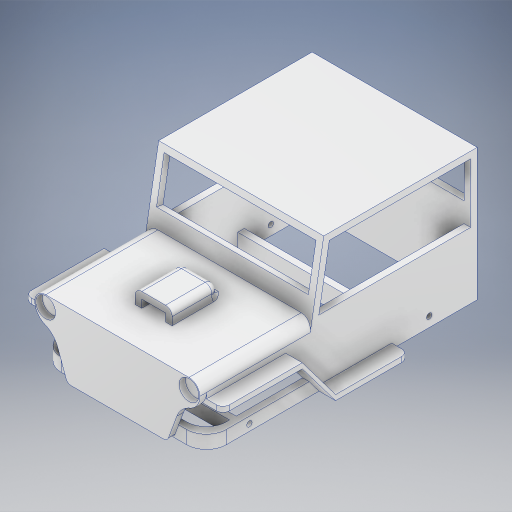
# Autodesk Inventor part: shell
Saved by Autodesk Inventor 2024 (Build 280153000, 153)
## iProperties
Created: 2024-04-09
Part Number: shell
Material: Aluminum 6061
Document SubType Name: Modeling
Designer: Alex
Density: 2.7 g/cm^3
Appearance: Aluminum - Flat
Mass: 9349.95 g
Surface Area: 5768.37 cm^2
Volume: 3462.95 cm^3
Author: Alex
Autodesk Inventor part; units mm, degrees
sketch "Sketch1" plane through (0, 0, 0) normal (1, 0, 0) x (0, 1, 0)
  line L0 (0, 0) -> (100, 0)
  line L1 (100, 0) -> (100, -160)
  line L2 (100, -410) -> (0, -410)
  line L3 (0, -410) -> (0, -400) construction
  line L4 (0, -410) -> (0, -410) construction
  line L5 (200, -410) -> (200, -177.6327)
  line L6 (200, -160) -> (100, -160) construction
  line L7 (100, -160) -> (0, -160) construction
  line L8 (100, -160) -> (100, -410) construction
  circle A0 centre (0, -50) radius 60 construction
  arc A1 (0, -400) -> (0, -280) centre (0, -340) ccw
  line L9 (0, -410) -> (24.2501, -410)
  line L10 (0, -393.7256) -> (0, -400)
  line L11 (0, -400) -> (0, -410)
  line L12 (0, -410) -> (200, -410)
  line L13 (0, -400) -> (0, -410)
  line L14 (0, -400) -> (0, 0) construction
  line L15 (0, -400) -> (0, -410)
  arc A2 (0, -400) -> (0, -400) centre (0, -340) ccw construction
  arc A3 (0, -280) -> (0, -400) centre (0, -340) ccw construction
  line L16 (0, -280) -> (0, -400) construction
  line L17 (0, -110) -> (0, -280)
  line L18 (75, 0) -> (67, 0)
  line L19 (67, 0) -> (67, -120)
  line L20 (67, -120) -> (75, -120) construction
  line L21 (75, -120) -> (75, 0)
  line L22 (8, -170.5357) -> (0, -170.5357) construction
  line L23 (0, -170.5357) -> (0, -280)
  line L24 (0, -280.5357) -> (8, -280.5357) construction
  line L25 (8, -280.5357) -> (8, -170.5357)
  line L26 (75, -120) -> (8, -170.5357)
  line L27 (67, -120) -> (0, -170.5357)
  line L28 (0, -280) -> (0, -280.5357) construction
  line L29 (100, -160) -> (200, -177.6327)
  line L30 (200, -177.6327) -> (200, -160) construction
  point P0 (67, 0)
  point P1 (0, -170.5357)
  dimension "d5" = 120
  dimension "d0" = 100
  dimension "d1" = 410
  dimension "d2" = 200
  dimension "d3" = 250
  dimension "d4" = 50
  dimension "d6" = 70
  dimension "d8" = 8
  dimension "d9" = 8
  dimension "d12" = 25
  dimension "d13" = 110
  dimension "d14" = 120
  dimension "d25" = 10
  dimension "d41" = 10
  constraints: 62 end point, 18 parallel, 10 perpendicular, 7 point on circle, 6 horizontal, 6 point on line, 3 centre point, 3 collinear, 1 midpoint, 1 vertical alignment, 3 other
  measures "d0" distance of L2.start L2.end
  measures "d1" distance of L0.end L2.start
  measures "d2" distance of L7.end L6.start
  measures "d3" distance of L6.start L5.start
  measures "d4" distance from line of point (0, -50) L0
  measures "d6" distance from line of L2 A1.centre
  measures "d8" distance of L19.end L20.end
  measures "d9" distance of L22.start L22.end
  measures "d12" distance between parallel lines of L21 L1
  measures "d13" distance of L24.end L22.start
  measures "d14" distance of L20.end L18.start
  measures "d25" angle of L29 L6
  measures "d41" distance of L11.start L4.end
extrude "Extrusion1" add sketch "Sketch1" against normal blind 250
sketch "Sketch2" plane through (0, 67, 0) normal (0, 0, 1) x (1, 0, 0)
  line L0 (-250, 33) -> (-250, 140.3403) projected
  line L1 (-250, 33) -> (0, 33)
  line L2 (0, 33) -> (0, -67) construction
  line L3 (-250, -67) -> (-250, 33) construction
  circle A0 centre (-233.5, 16.5) radius 15
  circle A1 centre (-16.5, 16.5) radius 15
  line L4 (0, 33) -> (0, 0) construction
  line L5 (0, 33) -> (-250, 33) construction
  line L6 (-250, 0) -> (-250, 33) construction
  line L7 (0, 0) -> (-250, 0) construction
  line L8 (-250, 16.5) -> (0, 16.5) construction
  arc A2 (-233.5, 33) -> (-250, 16.5) centre (-233.5, 16.5) ccw
  line L9 (0, 33) -> (-250, 33) projected
  line L10 (-250, 0) -> (-250, 33) projected
  arc A3 (0, 16.5) -> (-16.5, 33) centre (-16.5, 16.5) ccw
  line L11 (0, 33) -> (0, 0) projected
  arc A4 (-250, 16.5) -> (-234.6174, -6.5761) centre (-225, 16.5) ccw
  arc A5 (-215.1925, -26.9119) -> (-234.6174, -6.5761) centre (-248.0818, -38.8826) ccw
  line L12 (-215.1925, -26.9119) -> (-202.5175, -61.7362)
  arc A6 (-202.5175, -61.7362) -> (-195, -67) centre (-195, -59) ccw
  line L13 (-195, -67) -> (-55, -67)
  arc A7 (-55, -67) -> (-47.4825, -61.7362) centre (-55, -59) ccw
  line L14 (-47.4825, -61.7362) -> (-34.8075, -26.9119)
  arc A8 (-15.3826, -6.5761) -> (-34.8075, -26.9119) centre (-1.9182, -38.8826) ccw
  arc A9 (-15.3826, -6.5761) -> (0, 16.5) centre (-25, 16.5) ccw
  line L15 (-125, 16.5) -> (-125, -67) construction
  line L16 (0, -67) -> (-250, -67) construction
  line L17 (-250, -67) -> (0, -67) construction
  line L18 (0, 0) -> (-250, 0) projected
  line L19 (-6.2184, 0) -> (0, 0)
  line L20 (0, 0) -> (0, 16.5)
  line L21 (-243.7816, 0) -> (-250, 0)
  line L22 (-250, 0) -> (-250, 16.5)
  dimension "d17" = 30
  dimension "d18" = 25
  dimension "d19" = 8
  dimension "d20" = 35
  dimension "d21" = 140
  dimension "d22" = 110
  constraints: 26 end point, 18 point on circle, 16 tangent, 10 centre point, 6 point on line, 5 collinear, 5 midpoint, 4 equal radius, 2 concentric, 2 horizontal, 2 perpendicular, 1 equal length, 1 parallel, 1 vertical
  measures "d17" diameter of A1
  measures "d18" radius of A4
  measures "d19" radius of A6
  measures "d20" radius of A5
  measures "d21" distance of L13.start L13.end
  measures "d22" angle of L13 L12
extrude "Extrusion2" add sketch "Sketch2" along normal blind 10 contours L1 A3 A9 L18 A4 A2 | L18 A9 A8 L14 A7 L13 A6 L12 A5 A4
extrude "Extrusion3" cut sketch "Sketch2" against normal up to surface contours L1 A2 L10 | L1 L11 A3 surface through (0, 100, -160) normal (0, 0.1736482, 0.9848078)
extrude "Extrusion4" add sketch "Sketch1" along normal blind 25 contours L0 L21 L26 L25 A1 L17 L27 L19
ref_plane "Work Plane1" through (-125, 0, 0) normal (-1, 0, 0) x (0, 0, 1)
mirror "Mirror1" about plane through (-125, 0, 0) normal (-1, 0, 0) of "Extrusion4"
sketch "Sketch5" plane through (-125, 0, 0) normal (-1, 0, 0) x (0, 0, 1)
  line L0 (-120, 75) -> (0, 75) construction
  line L1 (0, 75) -> (0, 83.5) construction
  line L2 (-157.0906, 83.5) -> (0, 83.5) construction
  line L3 (-157.0906, 83.5) -> (-177.6327, 200) construction
  line L4 (-177.6327, 200) -> (-410, 200) construction
  line L5 (-410, 200) -> (-410, 0) construction
  line L6 (-410, 0) -> (-400, 0) construction
  arc A0 (-280.5357, 8) -> (-400, 0) centre (-340, 0) ccw construction
  line L7 (-280.5357, 8) -> (-170.5357, 8) construction
  line L8 (-170.5357, 8) -> (-120, 75) construction
  line L9 (-186.0237, 190) -> (-167.2449, 83.5)
  line L10 (-186.0237, 190) -> (-400, 190)
  line L11 (-400, 190) -> (-400, 0)
  line L12 (-157.0906, 83.5) -> (-410, 83.5) construction
  line L13 (-167.2449, 83.5) -> (-120, 83.5)
  line L14 (-157.0906, 83.5) -> (0, 83.5) construction
  line L15 (-120, 67) -> (-170.5357, 0) construction
  line L16 (-120, 67) -> (-170.5357, 0) construction
  line L17 (-120, 67) -> (-120, 83.5)
  line L18 (-120, 67) -> (-170.5357, 0) projected
  line L19 (-120, 67) -> (-170.5357, 0)
  line L20 (-170.5357, 0) -> (-280, 0)
  line L21 (-400, 0) -> (-400, 0)
  arc A1 (-280, 0) -> (-400, 0) centre (-340, 0) ccw
  point P0 (0, 0)
  dimension "d38" = 10
  dimension "d39" = 10
  dimension "d40" = 10
  constraints: 18 end point, 4 point on line, 3 collinear, 3 parallel, 2 point on circle, 1 centre point, 1 concentric, 1 vertical
  measures "d38" distance between parallel lines of L4 L10
  measures "d39" distance between parallel lines of L5 L11
  measures "d40" distance between parallel lines of L3 L9
extrude "Extrusion7" cut sketch "Sketch5" along normal mid plane 230
sketch "Sketch6" plane through (0, 0, 0) normal (1, 0, 0) x (0, 0, -1)
  line L0 (170.5357, 8) -> (280.5357, 8) construction
  arc A0 (400, 0) -> (280.5357, 8) centre (340, 0) ccw construction
  line L1 (400, 0) -> (410, 0) construction
  line L2 (410, 0) -> (410, 200) construction
  line L3 (410, 200) -> (177.6327, 200) construction
  line L4 (177.6327, 200) -> (157.0906, 83.5) construction
  line L5 (157.0906, 83.5) -> (0, 83.5) construction
  line L6 (0, 83.5) -> (0, 75) construction
  line L7 (0, 75) -> (120, 75) construction
  line L8 (120, 75) -> (170.5357, 8) construction
  line L9 (160, 100) -> (-10, 100) construction
  line L10 (170.1543, 100) -> (186.0237, 190)
  line L11 (186.0237, 190) -> (400, 190)
  line L12 (400, 190) -> (400, 100)
  line L13 (177.6327, 200) -> (157.0906, 83.5) projected
  line L14 (410, 200) -> (177.6327, 200) projected
  line L15 (410, 0) -> (410, 200) projected
  line L16 (170.1543, 100) -> (400, 100)
  point P0 (0, 0)
  dimension "d44" = 10
  dimension "d45" = 10
  dimension "d46" = 10
  dimension "d47" = 90
  constraints: 8 end point, 3 parallel, 2 horizontal
  measures "d44" distance between parallel lines of L10 L4
  measures "d45" distance between parallel lines of L11 L3
  measures "d46" distance between parallel lines of L2 L12
  measures "d47" distance between parallel lines of L11 L16
extrude "Extrusion8" cut sketch "Sketch6" against normal through all
sketch "Sketch7" plane through (-250, 200, -177.6327) normal (0, 0.1736482, 0.9848078) x (1, 0, 0)
  line L0 (250, 0) -> (250, -118.2972) construction
  line L1 (250, 0) -> (0, 0) construction
  line L2 (0, -118.2972) -> (0, 0) construction
  ellipse E0 centre (16.5, -118.2972) end of major axis (16.5, -135.0517) minor radius 16.5 (16.5, -101.5427) -> (0, -118.2972) ccw construction
  line L3 (233.5, -101.5427) -> (16.5, -101.5427) construction
  ellipse E1 centre (233.5, -118.2972) end of major axis (233.5, -101.5427) minor radius 16.5 (250, -118.2972) -> (233.5, -101.5427) ccw construction
  line L4 (10, -10) -> (240, -10)
  line L5 (240, -10) -> (240, -76.5427)
  line L6 (240, -76.5427) -> (10, -76.5427)
  line L7 (10, -76.5427) -> (10, -10)
  point P0 (250, -227.8071)
  dimension "d50" = 10
  dimension "d51" = 10
  dimension "d52" = 10
  dimension "d53" = 25
  constraints: 8 end point, 2 parallel, 1 horizontal, 1 perpendicular, 2 other
  measures "d50" distance between parallel lines of L0 L5
  measures "d51" distance between parallel lines of L2 L7
  measures "d52" distance between parallel lines of L4 L1
  measures "d53" distance between parallel lines of L3 L6
extrude "Extrusion9" cut sketch "Sketch7" against normal up to surface (10 mm away)
sketch "Sketch13" plane through (0, 0, 0) normal (1, 0, 0) x (0, 0, -1)
  arc A0 (400, 0) -> (280.5357, 8) centre (340, 0) ccw
  arc A1 (400, 0) -> (280.5357, 8) centre (340, 0) ccw projected
  line L0 (280, 0) -> (280.5357, 0)
  arc A2 (280, 0) -> (400, 0) centre (340, 0) ccw construction
  line L1 (170.5357, 0) -> (280, 0) construction
  line L2 (280, 0) -> (280, 8) construction
  arc A3 (400, 0) -> (280, 0) centre (340, 0) ccw projected
  line L3 (280, 8) -> (280.5357, 8) construction
  arc A4 (280.5357, 8) -> (280, 0) centre (340, 0) ccw construction
  line L4 (280.5357, 8) -> (280.5357, 0)
  line L5 (280.5357, 0) -> (400, 0)
  point P0 (0, 0)
  constraints: 10 end point, 6 point on circle, 3 centre point, 3 perpendicular, 3 tangent, 2 horizontal, 1 coincident, 1 concentric, 1 vertical
extrude "Extrusion11" add sketch "Sketch13" against normal blind 10
ref_plane "Work Plane2" through (-125, 0, 0) normal (1, 0, 0) x (0, 0, -1)
mirror "Mirror2" about plane through (-125, 0, 0) normal (1, 0, 0) of "Extrusion11"
sketch "Sketch15" plane through (-275, 67, 0) normal (-1, 0, 0) x (0, 0, 1)
  line L0 (-120, 8) -> (0, 8) construction
  line L1 (-170.5357, -59) -> (-120, 8) construction
  line L2 (-280.5357, -59) -> (-170.5357, -59) construction
  arc A0 (-280, -67) -> (-280.5357, -59) centre (-340, -67) ccw projected
  line L3 (-170.5357, -67) -> (-280, -67) construction
  line L4 (-120, 0) -> (-170.5357, -67) construction
  line L5 (0, 0) -> (-120, 0) construction
  line L6 (0, 8) -> (0, 0) construction
  line L7 (-280.5357, -59) -> (-280.5357, -67)
  line L8 (-280.5357, -67) -> (-280, -67)
  point P0 (0, -67)
  constraints: 4 end point, 1 perpendicular, 1 vertical
extrude "Extrusion12" add sketch "Sketch15" against normal up to surface (25 mm away)
mirror "Mirror3" about plane through (-125, 0, 0) normal (1, 0, 0) of "Extrusion12"
fillet "Fillet1" radius 10 1 edges at (-275, 4, -280.5357)
fillet "Fillet2" radius 10 1 edges at (25, 4, -280.5357)
sketch "Sketch16" plane through (0, 0, 0) normal (1, 0, 0) x (0, 0, -1)
  line L0 (280.5357, 8) -> (280.5357, 0) construction
  line L1 (280.5357, 0) -> (410, 0) construction
  line L2 (410, 0) -> (410, 200) construction
  line L3 (410, 200) -> (177.6327, 200) construction
  line L4 (177.6327, 200) -> (157.0906, 83.5) construction
  line L5 (157.0906, 83.5) -> (0, 83.5) construction
  line L6 (0, 83.5) -> (0, 75) construction
  line L7 (0, 75) -> (120, 75) construction
  line L8 (120, 75) -> (170.5357, 8) construction
  line L9 (170.5357, 8) -> (280.5357, 8) construction
  line L10 (186.0237, 190) -> (400, 190) construction
  line L11 (400, 190) -> (400, 100) construction
  line L12 (400, 100) -> (170.1543, 100) construction
  line L13 (170.1543, 100) -> (186.0237, 190) construction
  circle A0 centre (337.3259, 15) radius 4
  point P0 (0, 0)
  dimension "d70" = 8
  dimension "d71" = 15
  constraints: 1 centre point
  measures "d70" diameter of A0
  measures "d71" distance from line of L1 A0.centre
extrude "Extrusion13" cut sketch "Sketch16" against normal through all
fillet "Fillet3" radius 10 1 edges at (25, 71, 0)
fillet "Fillet4" radius 10 1 edges at (-275, 71, 0)
sketch "Sketch19" plane through (-10, 0, 0) normal (-1, 0, 0) x (0, 0, 1)
  line L0 (0, 40.0881) -> (0, 5.2638) projected
  line L1 (-170.5357, 0) -> (0, 0)
  line L2 (0, 0) -> (0, 20)
  line L3 (0, 20) -> (-170.5357, 20)
  line L4 (-170.5357, 20) -> (-170.5357, 0)
  line L5 (-120, 67) -> (-170.5357, 0) projected
  line L6 (-170.5357, 0) -> (-155.4504, 20)
  point P0 (0, 0)
  point P1 (0, 5.2638)
  dimension "d80" = 20
  constraints: 10 end point, 3 point on line, 2 parallel, 1 horizontal, 1 perpendicular
  measures "d80" distance of L2.end L1.end
extrude "Extrusion15" add sketch "Sketch19" against normal blind 10
mirror "Mirror5" about plane through (-125, 0, 0) normal (1, 0, 0) of "Extrusion15"
sketch "Sketch20" plane through (-10, 0, 0) normal (-1, 0, 0) x (0, 0, 1)
  line L0 (-155.4504, 20) -> (0, 20) projected
  line L1 (0, 0) -> (-10, 0)
  line L2 (-10, 0) -> (-10, 20)
  line L3 (-10, 20) -> (0, 20)
  line L4 (0, 20) -> (0, 0)
  dimension "d83" = 10
  constraints: 8 end point, 2 parallel, 1 horizontal, 1 perpendicular, 1 point on line
  measures "d83" distance between parallel lines of L4 L2
extrude "Extrusion16" add sketch "Sketch20" along normal up to surface (230 mm away)
fillet "Fillet5" radius 30 4 edges at (-10, 10, -10) (-240, 10, -10) (-250, 10, 0) (0, 10, 0)
sketch "Sketch21" plane through (0, 0, 0) normal (1, 0, 0) x (0, 0, -1)
  circle A0 centre (65, 10) radius 4
  line L0 (30, 0) -> (30, 20) construction
  line L1 (30, 0) -> (170.5357, 0) construction
  line L2 (155.4504, 20) -> (170.5357, 0) construction
  line L3 (155.4504, 20) -> (30, 20) construction
  line L4 (10, 67) -> (0, 67) construction
  line L5 (10, 67) -> (120, 67) construction
  line L6 (10, 67) -> (120, 67) construction
  line L7 (0, 67) -> (10, 67) construction
  line L8 (65, 67) -> (65, 0) construction
  line L9 (30, 0) -> (30, 20) construction
  line L10 (30, 10) -> (162.9931, 10) construction
  point P0 (0, 0)
  dimension "d87" = 8
  constraints: 4 end point, 3 midpoint, 3 point on line, 1 centre point, 1 perpendicular
  measures "d87" diameter of A0
extrude "Extrusion17" cut sketch "Sketch21" against normal through all
sketch "Sketch26" plane through (-240, 0, 0) normal (1, 0, 0) x (0, 0, -1)
  line L0 (40, 20) -> (10, 20) projected
  circle A0 centre (65, 10) radius 4 projected
  line L1 (40, 20) -> (155.4504, 20) projected
  line L2 (400, 0) -> (40, 0) projected
  line L3 (55, 20) -> (45, 20)
  line L4 (45, 20) -> (45, 0)
  line L5 (45, 0) -> (55, 0)
  line L6 (55, 0) -> (55, 20)
  point P0 (0, 0)
  dimension "d97" = 10
  dimension "d98" = 10
  constraints: 8 end point, 2 parallel, 2 point on line, 1 horizontal, 1 perpendicular
  measures "d97" distance of L5.end L4.end
  measures "d98" distance from line of L6 A0.centre
extrude "Extrusion19" add sketch "Sketch26" along normal up to surface (230 mm away) contours L1 L6 L2 L4
sketch "Sketch25" plane through (0, 67, 0) normal (0, 0, -1) x (-1, 0, 0)
  line L0 (42.1189, -47) -> (207.8811, -47) construction
  line L1 (215.1925, -26.9119) -> (207.8811, -47) construction
  arc A0 (234.6174, -6.5761) -> (215.1925, -26.9119) centre (248.0818, -38.8826) ccw construction
  arc A1 (234.6174, -6.5761) -> (243.7816, 0) centre (225, 16.5) ccw construction
  line L2 (6.2184, 0) -> (243.7816, 0) construction
  arc A2 (6.2184, 0) -> (15.3826, -6.5761) centre (25, 16.5) ccw construction
  arc A3 (34.8075, -26.9119) -> (15.3826, -6.5761) centre (1.9182, -38.8826) ccw construction
  line L3 (42.1189, -47) -> (34.8075, -26.9119) construction
  line L4 (125, 0) -> (125, -47) construction
  line L5 (33.3567, -23.5) -> (216.6433, -23.5) construction
  line L6 (85, -47) -> (57.5, 0)
  line L7 (165, -47) -> (192.5, 0)
  line L8 (85, -47) -> (165, -47)
  line L9 (125, -44.5) -> (125, -47) construction
  arc A4 (85, -47) -> (165, -47) centre (125, -23.5957) ccw construction
  line L10 (57.5, 0) -> (192.5, 0) construction
  line L11 (57.5, 0) -> (192.5, 0)
  point P0 (0, -67)
  dimension "d92" = 80
  dimension "d106" = 135
  constraints: 16 end point, 5 point on line, 4 point on circle, 3 collinear, 3 midpoint, 1 centre point, 1 coincident, 1 equal length, 1 horizontal, 1 tangent, 1 vertical
  measures "d92" distance of L6.start L7.start
  measures "d106" distance of L6.end L7.end
extrude "Extrusion18" add sketch "Sketch25" along normal up to surface (55 mm away)
ref_plane "Work Plane11" through (0, 67, -120) normal (0, -0.1045285, -0.9945219) x (1, 0, 0)
ref_plane "Work Plane12" through (-85, 20, 0) normal (0, -0.1045285, -0.9945219) x (1, 0, 0)
sketch "Sketch30" plane through (-85, 20, 0) normal (0, -0.1045285, -0.9945219) x (1, 0, 0)
  circle A0 centre (-40, -30.2876) radius 21
  point P0 (85, 19.8904)
  dimension "d114" = 42
  constraints: 1 centre point, 1 coincident, 1 other
  measures "d114" diameter of A0
extrude "Extrusion22" cut sketch "Sketch30" along normal up to surface surface through (-240, 0, -55) normal (0, 0, -1)
sketch "Sketch31" plane through (-125, 0, 0) normal (1, 0, 0) x (0, 0, -1)
  line L0 (0.9708, 29.2367) -> (5.361, 71.0066) construction
  line L1 (3.1659, 50.1216) -> (410, 7.3616) construction
  line L2 (400, 190) -> (186.0237, 190) construction
  line L3 (186.0237, 190) -> (170.1543, 100) construction
  line L4 (170.1543, 100) -> (400, 100) construction
  line L5 (400, 100) -> (400, 190) construction
  line L6 (170.5357, 8) -> (120, 75) construction
  line L7 (120, 75) -> (0, 75) construction
  line L8 (0, 75) -> (0, 83.5) construction
  line L9 (157.0906, 83.5) -> (0, 83.5) construction
  line L10 (157.0906, 83.5) -> (177.6327, 200) construction
  line L11 (177.6327, 200) -> (410, 200) construction
  line L12 (410, 200) -> (410, 0) construction
  line L13 (410, 0) -> (280.5357, 0) construction
  line L14 (280.5357, 0) -> (280.5357, 8) construction
  line L15 (280.5357, 8) -> (170.5357, 8) construction
  circle A0 centre (337.3259, 15) radius 4 construction
  line L16 (337.3259, 15) -> (297.3259, 15) construction
  line L17 (297.3259, 15) -> (297.3259, 19.2042) construction
  line L18 (297.3259, 30) -> (287.3259, 30)
  line L19 (287.3259, 30) -> (287.3259, 0)
  line L20 (287.3259, 0) -> (297.3259, 0)
  line L21 (297.3259, 0) -> (297.3259, 30)
  point P0 (0, 0)
  dimension "d118" = 40
  dimension "d119" = 10
  dimension "d120" = 30
  constraints: 14 end point, 4 point on line, 3 perpendicular, 2 horizontal, 2 parallel, 1 coincident, 1 midpoint
  measures "d118" distance of L16.start L16.end
  measures "d119" distance of L20.end L19.end
  measures "d120" distance of L19.end L18.end
extrude "Extrusion23" add sketch "Sketch31" along normal mid plane 230
ref_plane "Work Plane15" through (-125, 19.2042, -297.3259) normal (0, -0.1045285, -0.9945219) x (1, 0, 0)
sketch "Sketch34" plane through (-125, 19.2042, -297.3259) normal (0, -0.1045285, -0.9945219) x (1, 0, 0)
  circle A0 centre (0, 0) radius 4
  point P0 (125, 50.178)
  dimension "d126" = 8
  constraints: 1 centre point, 1 coincident
  measures "d126" diameter of A0
extrude "Extrusion25" cut sketch "Sketch34" along normal blind 5 and the other way blind 15
sketch "Sketch35" plane through (-233.5, 100, 10) normal (0, 1, 0) x (1, 0, 0)
  line L0 (0, 170) -> (0, 0) construction
  line L1 (217, 0) -> (0, 0) construction
  line L2 (217, 170) -> (217, 0) construction
  line L3 (217, 170) -> (0, 170) construction
  line L4 (90.5, 115) -> (126.5, 115)
  line L5 (126.5, 115) -> (126.5, 55)
  line L6 (126.5, 55) -> (90.5, 55)
  line L7 (90.5, 55) -> (90.5, 115)
  line L8 (0, 85) -> (217, 85) construction
  line L9 (217, 170) -> (0, 170) construction
  line L10 (108.5, 170) -> (108.5, 0) construction
  line L11 (90.5, 115) -> (126.5, 55) construction
  line L12 (90.5, 55) -> (126.5, 115) construction
  line L13 (80.5, 55) -> (80.5, 125)
  line L14 (80.5, 125) -> (136.5, 125)
  line L15 (136.5, 125) -> (136.5, 55)
  line L16 (80.5, 55) -> (90.5, 55)
  line L17 (136.5, 55) -> (126.5, 55)
  point P0 (233.5, 10)
  point P1 (108.5, 85)
  point P2 (108.5, 85)
  dimension "d131" = 60
  dimension "d132" = 36
  dimension "d133" = 10
  dimension "d134" = 10
  constraints: 26 end point, 7 midpoint, 4 parallel, 3 horizontal, 1 perpendicular, 1 vertical, 1 other
  measures "d131" distance of L4.end L5.end
  measures "d132" distance of L5.end L6.end
  measures "d133" distance between parallel lines of L7 L13
  measures "d134" distance between parallel lines of L4 L14
extrude "Extrusion26" add sketch "Sketch35" along normal blind 22
extrude "Extrusion27" cut sketch "Sketch35" along normal blind 12 contours L4 L5 L6 L7
fillet "Fillet6" radius 10 2 edges at (-125, 122, -115) (-125, 100, -115)
fillet "Fillet7" radius 10 8 edges at (-153, 119.0711, -112.0711) (-153, 111, -115) (-153, 102.9289, -117.9289) (-153, 122, -75) (-97, 119.0711, -112.0711) (-97, 111, -115) (-97, 102.9289, -117.9289) (-97, 122, -75)
sketch "Sketch37" plane through (0, 0, -410) normal (0, 0, -1) x (-1, 0, 0)
  line L0 (10, 190) -> (240, 190)
  line L1 (240, 190) -> (240, 130)
  line L2 (240, 130) -> (10, 130)
  line L3 (10, 130) -> (10, 190)
  line L4 (0, 200) -> (250, 200) construction
  line L5 (0, 0) -> (0, 200) construction
  line L6 (250, 200) -> (250, 0) construction
  dimension "d141" = 10
  dimension "d142" = 10
  dimension "d143" = 10
  dimension "d144" = 60
  constraints: 8 end point, 2 parallel, 1 horizontal, 1 perpendicular
  measures "d141" distance between parallel lines of L5 L3
  measures "d142" distance between parallel lines of L6 L1
  measures "d143" distance between parallel lines of L4 L0
  measures "d144" distance between parallel lines of L2 L0
extrude "Extrusion28" cut sketch "Sketch37" against normal up to surface (10 mm away)
equation "\"d9\" = d8"
equation "\"d39\" = d38"
equation "\"d40\" = d38"
equation "\"d45\" = d44"
equation "\"d46\" = d44"
equation "\"d51\" = d50"
equation "\"d52\" = d50"
body "Solid1"
